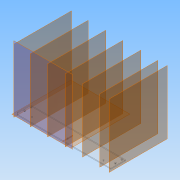
# Autodesk Inventor part: Pancake_Tilted Tube Backboard Long
Saved by Autodesk Inventor 2018.1 (Build 221171000, 171)
## iProperties
Created: 2019-02-21
Part Number: Pancake_Tilted Tube Backboard Long
Material: PET Plastic
Document SubType Name: Modeling
Designer: James
Density: 1.541 g/cm^3
Appearance: Polycarbonate - Clear
Author: James
Autodesk Inventor part; units mm, degrees
ref_plane "YZ Plane" through (0, 0, 0) normal (1, 0, 0) x (0, 1, 0)
ref_plane "XZ Plane" through (0, 0, 0) normal (0, 1, 0) x (-1, 0, 0)
ref_plane "XY Plane" through (0, 0, 0) normal (0, 0, 1) x (1, 0, 0)
derived "Pancake_Skeleton.ipt"
ref_plane "Ground" through (0, 0, 0) normal (0, 1, 0) x (-1, 0, 0)
ref_plane "Back" through (0, 0, 0) normal (0, 0, 1) x (1, 0, 0)
ref_plane "LHS" through (0, 0, 0) normal (1, 0, 0) x (0, 1, 0)
ref_plane "Lane 1" through (90, 0, 0) normal (1, 0, 0) x (0, 1, 0)
ref_plane "Lane 2" through (185, 0, 0) normal (1, 0, 0) x (0, 1, 0)
ref_plane "Lane 3" through (280, 0, 0) normal (1, 0, 0) x (0, 1, 0)
ref_plane "Lane 4" through (375, 0, 0) normal (1, 0, 0) x (0, 1, 0)
ref_plane "Lane 5" through (470, 0, 0) normal (1, 0, 0) x (0, 1, 0)
ref_plane "RHS" through (520, 0, 0) normal (1, 0, 0) x (0, 1, 0)
sketch "Sketch1" plane through (0, 0, 0) normal (0, 0, 1) x (1, 0, 0)
  line L0 (0, 96) -> (0, -16) projected
  line L1 (-104, 0) -> (624, 0) projected
  line L2 (520, 96) -> (520, -16) projected
  line L3 (0, 0) -> (520, 0)
  line L4 (520, 0) -> (520, 80)
  line L5 (520, 80) -> (0, 80)
  line L6 (0, 80) -> (0, 0)
  dimension "d1" = 80
  constraints: 8 end point, 2 parallel, 1 horizontal, 1 perpendicular, 1 point on line
  measures "d1" distance of L3.end L4.end
extrude "Extrusion1" add sketch "Sketch1" along normal blind 5
sketch "Sketch2" plane through (0, 0, 5) normal (0, 0, 1) x (1, 0, 0)
  line L0 (90, 96) -> (90, -16) projected
  line L1 (-104, 0) -> (624, 0) projected
  line L2 (520, 80) -> (0, 80) projected
  point P0 (0, 0)
  point P1 (90, 25)
  point P2 (90, 55)
  dimension "d4" = 30
  dimension "d5" = 25
  dimension "d6" = 25
  constraints: 1 point on line, 1 vertical alignment
  measures "d4" distance of point (90, 55) point (90, 25)
  measures "d5" distance from line of L1 point (90, 25)
  measures "d6" distance from line of L2 point (90, 55)
hole "Hole1" [suppressed]
sketch "Sketch3" plane through (0, 0, 5) normal (0, 0, 1) x (1, 0, 0)
  line L0 (0, 96) -> (0, -16) projected
  line L1 (520, 80) -> (0, 80) projected
  line L2 (-104, 0) -> (624, 0) projected
  point P0 (0, 0)
  point P1 (12.5, 72.5)
  point P2 (12.5, 37.5)
  dimension "d17" = 12.5
  dimension "d18" = 35
  dimension "d19" = 7.5
  dimension "d49" = 37.5
  constraints: 1 vertical alignment
  measures "d17" distance from line of point (12.5, 72.5) L0
  measures "d18" distance of point (12.5, 37.5) point (12.5, 72.5)
  measures "d19" distance from line of L1 point (12.5, 72.5)
  measures "d49" distance from line of L2 point (12.5, 37.5)
hole "Hole2" at (12.5, 72.5, 5) at (12.5, 37.5, 5) direction (0, 0, -1) diameter 4.5 end through all countersink diameter 9.4 countersink angle 90 clearance for "Flat Head Machine Screw" size "M4" standard "Ansi Metric M Profile"
ref_plane "Mid Plane" through (260, 0, 0) normal (-1, 0, 0) x (0, 0, 1)
mirror "Mirror1" about plane through (260, 0, 0) normal (-1, 0, 0) of "Hole2"
sketch "Sketch4" plane through (0, 0, 5) normal (0, 0, 1) x (1, 0, 0)
  line L0 (0, 96) -> (0, -16) projected
  line L1 (520, 96) -> (520, -16) projected
  line L2 (520, 80) -> (0, 80) projected
  line L3 (-104, 0) -> (624, 0) projected
  point P0 (0, 0)
  point P1 (60.0625, 30)
  point P2 (260, 25)
  point P3 (459.9375, 20)
  dimension "d28" = 5
  dimension "d29" = 5
  dimension "d34" = 55
  dimension "d35" = 25
  dimension "d43" = 200
  dimension "d44" = 200
  dimension "d47" = 60.0625
  dimension "d48" = 60.0625
  measures "d28" vertical distance of point (260, 25) point (60.063, 30)
  measures "d29" vertical distance of point (459.937, 20) point (260, 25)
  measures "d34" distance from line of L2 point (260, 25)
  measures "d35" distance from line of L3 point (260, 25)
  measures "d43" distance of point (260, 25) point (60.063, 30)
  measures "d44" distance of point (459.937, 20) point (260, 25)
  measures "d47" distance from line of L1 point (459.937, 20)
  measures "d48" distance from line of point (60.063, 30) L0
hole "Hole3" at (60.0625, 30, 5) at (260, 25, 5) at (459.9375, 20, 5) direction (0, 0, -1) diameter 4.5 end through all clearance for "Flat Head Machine Screw" size "M4" standard "Ansi Metric M Profile"
chamfer "Chamfer1" distance 10 angle 45 1 edges at (0, 0, 2.5)
equation "\"d5\" = d6"
equation "\"d29\" = d28"
equation "\"d44\" = d43"
equation "\"d47\" = d48"
body "Solid1"
